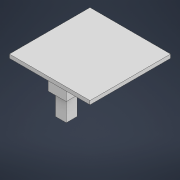
# Autodesk Inventor part: QRholderSpecial-top
Saved by Autodesk Inventor 2022 (Build 260153000, 153)
## iProperties
Created: 2023-05-03
Part Number: QRholderSpecial-top
Material: Všeobecné
Document SubType Name: Modeling
Designer: tada
Density: 1 g/cm^3
Appearance: Výchozí
Author: tada
Autodesk Inventor part; units mm, degrees
ref_plane "YZ Plane" through (0, 0, 0) normal (1, 0, 0) x (0, 1, 0)
ref_plane "XZ Plane" through (0, 0, 0) normal (0, 1, 0) x (-1, 0, 0)
ref_plane "XY Plane" through (0, 0, 0) normal (0, 0, 1) x (1, 0, 0)
sketch "Náčrt1" plane through (0, 0, 0) normal (0, 1, 0) x (-1, 0, 0)
  line L0 (0, 2.95) -> (-2.95, 2.95)
  line L1 (-2.95, 2.95) -> (-2.95, 0)
  line L2 (-2.95, 0) -> (0, 0)
  line L3 (0, 0) -> (0, 2.95)
  dimension "d0" = 2.95
  dimension "d1" = 2.95
  constraints: 8 end point, 2 parallel, 2 point on line, 1 horizontal, 1 perpendicular
  measures "d0" distance between parallel lines of L1 L3
  measures "d1" distance between parallel lines of L2 L0
extrude "Vysunutí1" add sketch "Náčrt1" along normal blind 6
sketch "Náčrt2" plane through (0, 6, 0) normal (0, 1, 0) x (1, 0, 0)
  line L0 (-1, -3.95) -> (3.95, -3.95)
  line L1 (3.95, -3.95) -> (3.95, 1)
  line L2 (3.95, 1) -> (-1, 1)
  line L3 (-1, 1) -> (-1, -3.95)
  line L4 (0, 0) -> (0, -2.95) projected
  line L5 (0, -2.95) -> (2.95, -2.95) projected
  line L6 (2.95, -2.95) -> (2.95, 0) projected
  line L7 (2.95, 0) -> (0, 0) projected
  dimension "d4" = 1
  dimension "d5" = 1
  dimension "d6" = 1
  dimension "d7" = 1
  constraints: 8 end point, 2 parallel, 1 horizontal, 1 perpendicular
  measures "d4" distance between parallel lines of L3 L4
  measures "d5" distance between parallel lines of L0 L5
  measures "d6" distance between parallel lines of L6 L1
  measures "d7" distance between parallel lines of L2 L7
extrude "Vysunutí2" add sketch "Náčrt2" along normal blind 10 contours L3 L2 L1 L0 | L7 L6 L5 L4
sketch "Náčrt3" plane through (0, 16, 0) normal (0, 1, 0) x (1, 0, 0)
  line L0 (-4.05, 10.525) -> (17.95, 10.525)
  line L1 (17.95, 10.525) -> (17.95, -11.475)
  line L2 (17.95, -11.475) -> (-4.05, -11.475)
  line L3 (-4.05, -11.475) -> (-4.05, 10.525)
  line L4 (3.95, -3.95) -> (3.95, 1) projected
  line L5 (-1, -3.95) -> (3.95, -3.95) projected
  line L6 (3.95, 1) -> (-1, 1) projected
  line L7 (-1, 1) -> (-1, -3.95) projected
  point P0 (0, 0)
  dimension "d10" = 14
  dimension "d11" = 22
  dimension "d12" = 22
  dimension "d13" = 9.525
  dimension "d14" = 7.525
  dimension "d17" = 3.05
  constraints: 8 end point, 2 parallel, 1 horizontal, 1 perpendicular
  measures "d10" distance between parallel lines of L1 L4
  measures "d11" distance between parallel lines of L3 L1
  measures "d12" distance between parallel lines of L2 L0
  measures "d13" distance between parallel lines of L0 L6
  measures "d14" distance between parallel lines of L2 L5
  measures "d17" distance between parallel lines of L7 L3
extrude "Vysunutí3" add sketch "Náčrt3" along normal blind 1 contours L0 L1 L2 L3 | L5 L7 L6 L4
equation "\"d1\" = d0"
equation "\"d5\" = d4"
equation "\"d6\" = d4"
equation "\"d7\" = d4"
equation "\"d12\" = d11"
